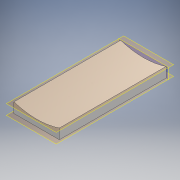
# Autodesk Inventor part: 2.2.1SujayPrototype
Saved by Autodesk Inventor 2018 (Build 220112000, 112)
## iProperties
Created: 2017-11-02
Part Number: 2.2.1SujayPrototype
Material: Generic
Document SubType Name: Modeling
Designer: 228924
Density: 1 g/cm^3
Appearance: Default
Author: 228924
Autodesk Inventor part; units mm, degrees
ref_plane "Work Plane1" through (0, -200, 0) normal (0, 1, 0) x (-1, 0, 0)
ref_plane "YZ Plane" through (0, 0, 0) normal (1, 0, 0) x (0, 1, 0)
ref_plane "Work Plane1" through (0, -200, 0) normal (0, 1, 0) x (-1, 0, 0)
sketch "Sketch1" plane through (0, -200, 0) normal (0, 1, 0) x (-1, 0, 0)
  line L0 (0, 0) -> (-85, 0)
  line L1 (-85, 0) -> (-85, 19)
  line L2 (0, 0) -> (0, 19)
  arc A0 (-85, 19) -> (0, 19) centre (-42.5, 147.1357) ccw
  dimension "d1" = 85
  dimension "d2" = 19
  dimension "d3" = 19
  dimension "d4" = 135
  constraints: 6 end point, 2 point on circle, 1 centre point, 1 horizontal, 1 perpendicular, 1 vertical
  measures "d1" distance of L0.start L0.end
  measures "d2" distance of L0.end L1.end
  measures "d3" distance of L0.start L2.end
  measures "d4" radius of A0
extrude "Extrusion1" add sketch "Sketch1" along normal blind 200
ref_plane "Work Plane3" through (0, 0, 19) normal (0, 0, 1) x (1, 0, 0)
body "Solid1"
